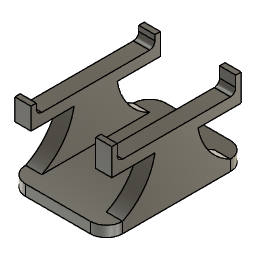
plane_stand_f3d (Autodesk Fusion 360 design; units mm, degrees)
Autodesk Fusion 360 part; units mm, degrees
note: some values were not read from the file. Set by a fixed rule: which sketch regions a step uses.
sketch "Sketch1" plane through (0, 0, 0) normal (0, 0, 1) x (1, 0, 0)
  line L0 (19.05, 0) -> (95.25, 0)
  line L1 (114.3, 19.05) -> (114.3, 146.05)
  line L2 (95.25, 165.1) -> (19.05, 165.1)
  line L3 (0, 146.05) -> (0, 19.05)
  arc A0 (0, 19.05) -> (19.05, 0) centre (19.05, 19.05) ccw
  arc A1 (95.25, 0) -> (114.3, 19.05) centre (95.25, 19.05) ccw
  arc A2 (19.05, 165.1) -> (0, 146.05) centre (19.05, 146.05) ccw
  arc A3 (114.3, 146.05) -> (95.25, 165.1) centre (95.25, 146.05) ccw
  point P0 (114.3, 0)
  point P1 (0, 165.1)
  dimension "d1" = 165.1
  dimension "d2" = 114.3
  dimension "d3" = 19.05
  dimension "d4" = 19.05
  dimension "d5" = 19.05
  dimension "d6" = 19.05
  constraint horizontal L0
  constraint vertical L1
  constraint horizontal L2
  constraint vertical L3
  constraint coincident origin L0
  constraint coincident origin L3
  constraint tangent L0 A0
  constraint tangent L3 A0
  constraint coincident P0 L0
  constraint coincident P0 L1
  constraint tangent L0 A1
  constraint tangent L1 A1
  constraint coincident P1 L2
  constraint coincident P1 L3
  constraint tangent L2 A2
  constraint tangent L3 A2
  constraint tangent L1 A3
  constraint tangent L2 A3
  measures "d1" distance of origin P1
  measures "d2" distance of origin P0
  measures "d3" radius of A0
  measures "d4" radius of A1
  measures "d5" radius of A2
  measures "d6" radius of A3
extrude "Extrude1" add sketch "Sketch1" along normal blind 12.7
sketch "Sketch2" plane through (0, 0, 12.7) normal (0, 0, 1) x (-1, 0, 0)
  arc A0 (-114.3, -146.05) -> (-95.25, -165.1) centre (-95.25, -146.05) ccw
  line L0 (-95.25, -165.1) -> (-19.05, -165.1)
  arc A1 (-19.05, -165.1) -> (0, -146.05) centre (-19.05, -146.05) ccw
  line L1 (0, -146.05) -> (0, -19.05)
  arc A2 (0, -19.05) -> (-19.05, 0) centre (-19.05, -19.05) ccw
  line L2 (-19.05, 0) -> (-95.25, 0)
  arc A3 (-95.25, 0) -> (-114.3, -19.05) centre (-95.25, -19.05) ccw
  line L3 (-114.3, -19.05) -> (-114.3, -146.05)
  line L4 (0, -146.05) -> (-19.05, -146.05)
  line L5 (-19.05, -146.05) -> (-19.05, -19.05)
  line L6 (-19.05, -19.05) -> (0, -19.05)
  line L7 (0, -19.05) -> (0, -146.05)
  line L8 (-95.25, -146.05) -> (-114.3, -146.05)
  line L9 (-114.3, -146.05) -> (-114.3, -19.05)
  line L10 (-114.3, -19.05) -> (-95.25, -19.05)
  line L11 (-95.25, -19.05) -> (-95.25, -146.05)
  constraint horizontal L4
  constraint vertical L5
  constraint horizontal L6
  constraint vertical L7
  constraint coincident A2.centre L5.end
  constraint coincident A1.end L1.start
  constraint horizontal L8
  constraint vertical L9
  constraint horizontal L10
  constraint vertical L11
  constraint coincident A3.end L3.start
  constraint coincident A0.centre L8.start
extrude "Extrude2" add sketch "Sketch2" along normal blind 76.2 contours L1 L4 L5 L6 L7
extrude "Extrude3" add sketch "Sketch2" along normal blind 76.2 contours L3 L8 L9 L10 L11
extrude "Extrude4" cut 1 faces at (12.7, 61.3833, 88.9) along direction (0, 0, -1) blind 25.4
extrude "Extrude5" cut 1 faces at (107.95, 103.7167, 88.9) along direction (0, 0, -1) blind 25.4
sketch "Sketch3" plane through (0, 0, 0) normal (-1, 0, 0) x (0, -1, 0)
  line L0 (-19.05, 63.5) -> (-146.05, 63.5)
  line L1 (-146.05, 63.5) -> (-146.05, 12.7)
  line L2 (-146.05, 12.7) -> (-146.05, 0)
  line L3 (-146.05, 0) -> (-19.05, 0)
  line L4 (-19.05, 0) -> (-19.05, 12.7)
  line L5 (-19.05, 12.7) -> (-19.05, 63.5)
  line L6 (-107.95, 63.5) -> (-57.15, 63.5)
  arc A0 (-146.05, 12.7) -> (-107.95, 63.5) centre (-176.7736, 75.4302) ccw
  arc A1 (-57.15, 63.5) -> (-19.05, 12.7) centre (11.6736, 75.4302) ccw
  point P0 (-82.55, 63.5)
  point P1 (-82.55, 63.5)
  dimension "d18" = 50.8
  dimension "d19" = 69.85
  dimension "d20" = 69.85
  constraint horizontal L6
  constraint midpoint L6 P1
  constraint midpoint L0 P1
  constraint coincident P1 P0
  constraint coincident L1.end L2.start
  constraint coincident L4.end L5.start
  measures "d18" distance of L6.start L6.end
  measures "d19" radius of A0
  measures "d20" radius of A1
extrude "Extrude6" cut sketch "Sketch3" against normal blind 200.66 contours L0 L5 A1 | L0 L1 A0
sketch "Sketch4" plane through (0, 0, 63.5) normal (0, 0, 1) x (-1, 0, 0)
  line L0 (-19.05, -107.95) -> (0, -107.95)
  line L1 (0, -107.95) -> (0, -57.15)
  line L2 (0, -57.15) -> (-19.05, -57.15)
  line L3 (-19.05, -57.15) -> (-19.05, -107.95)
  line L4 (0, -158.75) -> (-19.05, -158.75)
  line L5 (-19.05, -158.75) -> (-19.05, -6.35)
  line L6 (-19.05, -6.35) -> (0, -6.35)
  line L7 (0, -6.35) -> (0, -158.75)
  point P0 (0, -82.55)
  point P1 (0, -82.55)
  dimension "d29" = 19.05
  dimension "d30" = 152.4
  constraint midpoint L1 P1
  constraint horizontal L4
  constraint vertical L5
  constraint horizontal L6
  constraint vertical L7
  constraint midpoint L7 P1
  constraint coincident P1 P0
  measures "d29" distance of L4.start L4.end
  measures "d30" distance of L4.start L6.end
extrude "Extrude9" add sketch "Sketch4" along normal blind 12.7
sketch "Sketch5" plane through (0, 0, 63.5) normal (0, 0, 1) x (-1, 0, 0)
  line L0 (-114.3, -107.95) -> (-95.25, -107.95)
  line L1 (-95.25, -107.95) -> (-95.25, -57.15)
  line L2 (-95.25, -57.15) -> (-114.3, -57.15)
  line L3 (-114.3, -57.15) -> (-114.3, -107.95)
  line L4 (-95.25, -158.75) -> (-114.3, -158.75)
  line L5 (-114.3, -158.75) -> (-114.3, -6.35)
  line L6 (-114.3, -6.35) -> (-95.25, -6.35)
  line L7 (-95.25, -6.35) -> (-95.25, -158.75)
  point P0 (-114.3, -82.55)
  point P1 (-114.3, -82.55)
  dimension "d35" = 19.05
  dimension "d36" = 152.4
  constraint horizontal L4
  constraint vertical L5
  constraint horizontal L6
  constraint vertical L7
  constraint midpoint L3 P1
  constraint midpoint L5 P1
  constraint coincident P1 P0
  measures "d35" distance of L4.start L4.end
  measures "d36" distance of L4.end L5.end
extrude "Extrude10" add sketch "Sketch5" along normal blind 12.7
sketch "Sketch6" plane through (0, 0, 76.2) normal (0, 0, 1) x (-1, 0, 0)
  line L0 (0, -6.35) -> (-19.05, -6.35)
  line L1 (-19.05, -6.35) -> (-19.05, -158.75)
  line L2 (-19.05, -158.75) -> (0, -158.75)
  line L3 (0, -158.75) -> (0, -6.35)
  line L4 (-19.05, -6.35) -> (0, -6.35)
  line L5 (0, -6.35) -> (0, -19.05)
  line L6 (0, -19.05) -> (-19.05, -19.05)
  line L7 (-19.05, -19.05) -> (-19.05, -6.35)
  line L8 (0, -158.75) -> (-19.05, -158.75)
  line L9 (-19.05, -158.75) -> (-19.05, -146.05)
  line L10 (-19.05, -146.05) -> (0, -146.05)
  line L11 (0, -146.05) -> (0, -158.75)
  dimension "d39" = 12.7
  dimension "d40" = 12.7
  constraint horizontal L4
  constraint vertical L5
  constraint horizontal L6
  constraint vertical L7
  constraint coincident L3 L5.end
  constraint coincident L0.end L1.start
  constraint horizontal L8
  constraint vertical L9
  constraint horizontal L10
  constraint vertical L11
  constraint coincident L1 L9.end
  constraint coincident L2.end L3.start
  measures "d39" distance of L0.start L5.end
  measures "d40" distance of L2.end L10.end
extrude "Extrude11" add sketch "Sketch6" along normal blind 6.35 contours L0 L1 L3 L4 L5 L6 L7
extrude "Extrude12" add sketch "Sketch6" along normal blind 6.35 contours L1 L2 L3 L8 L9 L10 L11
sketch "Sketch7" plane through (0, 0, 76.2) normal (0, 0, 1) x (-1, 0, 0)
  line L0 (-95.25, -6.35) -> (-114.3, -6.35)
  line L1 (-114.3, -6.35) -> (-114.3, -158.75)
  line L2 (-114.3, -158.75) -> (-95.25, -158.75)
  line L3 (-95.25, -158.75) -> (-95.25, -6.35)
  line L4 (-114.3, -6.35) -> (-95.25, -6.35)
  line L5 (-95.25, -6.35) -> (-95.25, -19.05)
  line L6 (-95.25, -19.05) -> (-114.3, -19.05)
  line L7 (-114.3, -19.05) -> (-114.3, -6.35)
  line L8 (-95.25, -158.75) -> (-114.3, -158.75)
  line L9 (-114.3, -158.75) -> (-114.3, -146.05)
  line L10 (-114.3, -146.05) -> (-95.25, -146.05)
  line L11 (-95.25, -146.05) -> (-95.25, -158.75)
  dimension "d45" = 12.7
  dimension "d60" = 12.7
  constraint horizontal L4
  constraint vertical L5
  constraint horizontal L6
  constraint vertical L7
  constraint coincident L3 L5.end
  constraint coincident L0.end L1.start
  constraint horizontal L8
  constraint vertical L9
  constraint horizontal L10
  constraint vertical L11
  constraint coincident L1 L9.end
  constraint coincident L2.end L3.start
  measures "d45" distance of L0.end L6.end
  measures "d60" distance of L1.end L9.end
extrude "Extrude13" add sketch "Sketch7" along normal blind 6.35 contours L0 L1 L3 L4 L5 L6 L7 | L1 L2 L3 L8 L9 L10 L11
sketch "Sketch8" plane through (114.3, 0, 0) normal (1, 0, 0) x (0, 1, 0)
  arc A0 (107.95, 63.5) -> (146.05, 12.7) centre (176.7736, 75.4302) ccw
  line L0 (107.95, 63.5) -> (158.75, 63.5)
  line L1 (158.75, 63.5) -> (158.75, 82.55)
  line L2 (146.05, 76.2) -> (19.05, 76.2)
  line L3 (6.35, 82.55) -> (6.35, 63.5)
  line L4 (6.35, 63.5) -> (57.15, 63.5)
  arc A1 (19.05, 12.7) -> (57.15, 63.5) centre (-11.6736, 75.4302) ccw
  line L5 (19.05, 12.7) -> (19.05, 0)
  line L6 (19.05, 0) -> (146.05, 0)
  line L7 (146.05, 0) -> (146.05, 12.7)
  line L8 (158.75, 63.5) -> (158.75, 82.55)
  arc A2 (12.7, 82.55) -> (19.05, 76.2) centre (19.05, 82.55) ccw
  line L9 (6.35, 82.55) -> (12.7, 82.55)
  line L10 (152.4, 82.55) -> (158.75, 82.55)
  arc A3 (146.05, 76.2) -> (152.4, 82.55) centre (146.05, 82.55) ccw
  line L11 (12.7, 82.55) -> (19.05, 82.55)
  line L12 (19.05, 82.55) -> (19.05, 76.2)
  line L13 (146.05, 76.2) -> (146.05, 82.55)
  line L14 (146.05, 82.55) -> (152.4, 82.55)
  line L15 (146.05, 82.55) -> (146.05, 76.2)
  line L16 (19.05, 82.55) -> (6.35, 82.55)
  arc A4 (107.95, 63.5) -> (146.05, 12.7) centre (176.7736, 75.4302) ccw
  line L17 (107.95, 63.5) -> (158.75, 63.5)
  line L18 (146.05, 82.55) -> (146.05, 76.2)
  line L19 (146.05, 76.2) -> (19.05, 76.2)
  line L20 (19.05, 76.2) -> (19.05, 82.55)
  line L21 (19.05, 82.55) -> (6.35, 82.55)
  line L22 (6.35, 82.55) -> (6.35, 63.5)
  line L23 (6.35, 63.5) -> (57.15, 63.5)
  arc A5 (19.05, 12.7) -> (57.15, 63.5) centre (-11.6736, 75.4302) ccw
  line L24 (19.05, 12.7) -> (19.05, 0)
  line L25 (19.05, 0) -> (146.05, 0)
  line L26 (146.05, 0) -> (146.05, 12.7)
  point P0 (12.7, 82.55)
  point P1 (152.4, 82.55)
  dimension "d50" = 6.35
  dimension "d51" = 6.35
  dimension "d52" = 6.35
  dimension "d53" = 6.35
  constraint tangent L2 A2
  constraint coincident L2.end A2.end
  constraint coincident P0 A2.start
  constraint coincident L3.start L9.start
  constraint coincident P1 L10.start
  constraint coincident L1.end L8.end
  constraint perpendicular L8 L10
  constraint coincident L2.start A3.start
  constraint coincident A2.centre L11.end
  constraint coincident A3.centre L13.end
  measures "d50" distance of L3.start P0
  measures "d51" distance of P1 L1.end
  measures "d52" radius of A2
  measures "d53" radius of A3
extrude "Extrude14" cut sketch "Sketch8" against normal blind 147.32 contours A3 L13 L14 L15 L18 | A2 L11 L12 L16 L20 L21
extrude "Extrude15" add 1 faces at (6.35, 10.5833, 82.55) along direction (0, 0, 1) blind 6.35
extrude "Extrude16" add 1 faces at (101.6, 10.5833, 82.55) along direction (0, 0, 1) blind 6.35
extrude "Extrude17" add 1 faces at (101.6, 10.5833, 88.9) along direction (0, 0, 1) blind 6.35
extrude "Extrude18" add 1 faces at (6.35, 10.5833, 88.9) along direction (0, 0, 1) blind 6.35
extrude "Extrude19" cut 1 faces at (101.6, 10.5833, 95.25) along direction (0, 0, -1) blind 12.7
extrude "Extrude20" cut 1 faces at (6.35, 10.5833, 95.25) along direction (0, 0, -1) blind 12.7
extrude "Extrude21" add 1 faces at (101.6, 10.5833, 82.55) along direction (0, 0, 1) blind 12.7
extrude "Extrude22" add 1 faces at (101.6, 156.6333, 82.55) along direction (0, 0, 1) blind 12.7
extrude "Extrude23" add 1 faces at (12.7, 154.5167, 82.55) along direction (0, 0, 1) blind 6.35
extrude "Extrude24" add 1 faces at (6.35, 10.5833, 82.55) along direction (0, 0, 1) blind 6.35
equation "d4 = d3"
equation "d5 = d3"
equation "d6 = d3"
equation "d20 = d19"
equation "d40 = d39"
equation "d51 = d50"
equation "d53 = d52"
